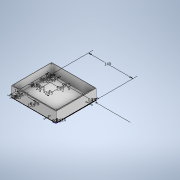
# Autodesk Inventor part: Couvercle inférieur
Saved by Autodesk Inventor 2020 (Build 240168000, 168)
## iProperties
Created: 2020-01-03
Part Number: Couvercle inférieur
Material: Générique
Document SubType Name: Modeling
Designer: Manuel Enzo
Density: 1 g/cm^3
Appearance: Par défaut
Author: Manuel Enzo
Autodesk Inventor part; units mm, degrees
ref_plane "YZ Plane" through (0, 0, 0) normal (1, 0, 0) x (0, 1, 0)
ref_plane "XZ Plane" through (0, 0, 0) normal (0, 1, 0) x (-1, 0, 0)
ref_plane "XY Plane" through (0, 0, 0) normal (0, 0, 1) x (1, 0, 0)
sketch "Esquisse1" plane through (0, 0, 0) normal (0, 1, 0) x (-1, 0, 0)
  line L0 (0, 0) -> (140, 0)
  line L1 (140, 0) -> (140, -126)
  line L2 (140, -126) -> (0, -126)
  line L3 (0, -126) -> (0, 0)
  line L4 (1, -1) -> (139, -1)
  line L5 (139, -1) -> (139, -125)
  line L6 (139, -125) -> (1, -125)
  line L7 (1, -125) -> (1, -1)
  line L8 (138, -2) -> (2, -2)
  line L9 (2, -2) -> (2, -124)
  line L10 (2, -124) -> (138, -124)
  line L11 (138, -124) -> (138, -2)
  circle A0 centre (135.5, -4.5) radius 2.5
  circle A1 centre (135.5, -4.5) radius 0.75
  circle A2 centre (135.5, -4.5) radius 1.5
  circle A3 centre (135.5, -121.5) radius 2.5
  circle A4 centre (135.5, -121.5) radius 1.5
  circle A5 centre (135.5, -121.5) radius 0.75
  circle A6 centre (4.5, -121.5) radius 2.5
  circle A7 centre (4.5, -121.5) radius 1.5
  circle A8 centre (4.5, -121.5) radius 0.75
  circle A9 centre (4.5, -4.5) radius 2.5
  circle A10 centre (4.5, -4.5) radius 1.5
  circle A11 centre (4.5, -4.5) radius 0.75
  circle A12 centre (135.25, -93.5) radius 2.5
  circle A13 centre (135.25, -93.5) radius 0.25
  circle A14 centre (87.25, -99.5) radius 2.5
  circle A15 centre (87.25, -99.5) radius 0.25
  circle A16 centre (135.25, -17.5) radius 2.5
  circle A17 centre (135.25, -17.5) radius 0.25
  circle A18 centre (87.25, -17.5) radius 2.5
  circle A19 centre (87.25, -17.5) radius 0.25
  circle A20 centre (119.75, -69) radius 2.5
  circle A21 centre (119.75, -69) radius 0.25
  circle A22 centre (91.75, -69) radius 2.5
  circle A23 centre (91.75, -69) radius 0.25
  point P0 (0, -11)
  point P1 (0, -19)
  point P2 (0, -26.5)
  point P3 (0, -34.5)
  point P4 (0, -40)
  point P5 (0, -49)
  point P6 (97.5, -53)
  point P7 (100, -50.5)
  point P8 (4.5, -2)
  point P9 (2, -4.5)
  point P10 (2, -121.5)
  point P11 (4.5, -124)
  point P12 (135.5, -124)
  point P13 (138, -121.5)
  point P14 (138, -4.5)
  point P15 (135.5, -2)
  dimension "d0" = 126
  dimension "d1" = 140
  dimension "d2" = 1
  dimension "d3" = 1
  dimension "d4" = 1
  dimension "d5" = 1
  dimension "d6" = 1
  dimension "d8" = 1
  dimension "d10" = 124
  dimension "d11" = 1
  dimension "d12" = 1
  dimension "d13" = 0.75
  dimension "d14" = 5
  dimension "d15" = 2.5
  dimension "d16" = 2.5
  dimension "d17" = 0.75
  dimension "d18" = 1
  dimension "d19" = 5
  dimension "d20" = 2.5
  dimension "d21" = 2.5
  dimension "d22" = 0.75
  dimension "d23" = 1
  dimension "d24" = 5
  dimension "d25" = 2.5
  dimension "d26" = 2.5
  dimension "d27" = 5
  dimension "d28" = 1
  dimension "d29" = 0.75
  dimension "d30" = 2.5
  dimension "d31" = 2.5
  dimension "d114" = 2.25
  dimension "d115" = 5
  dimension "d118" = 2.25
  dimension "d119" = 5
  dimension "d134" = 2.25
  dimension "d135" = 5
  dimension "d150" = 2.25
  dimension "d151" = 5
  dimension "d166" = 2.25
  dimension "d167" = 5
  dimension "d170" = 2.25
  dimension "d171" = 5
  dimension "d176" = 2.75
  dimension "d177" = 15.5
  dimension "d178" = 15.5
  dimension "d179" = 50.75
  dimension "d180" = 18.25
  dimension "d181" = 46.25
  dimension "d182" = 2.75
  dimension "d183" = 50.75
  dimension "d184" = 30.5
  dimension "d185" = 24.5
  dimension "d186" = 55
  dimension "d187" = 55
  constraints: 24 centre point, 24 end point, 14 coincident, 6 parallel, 3 horizontal, 3 perpendicular
  measures "d0" distance between parallel lines of L0 L2
  measures "d1" distance between parallel lines of L3 L1
  measures "d2" distance between parallel lines of L5 L11
  measures "d3" distance between parallel lines of L10 L6
  measures "d4" distance between parallel lines of L7 L9
  measures "d5" distance between parallel lines of L8 L4
  measures "d6" distance between parallel lines of L3 L7
  measures "d8" distance between parallel lines of L6 L2
  measures "d10" distance of L6.end L4.start
  measures "d11" distance between parallel lines of L1 L5
  measures "d12" radial gap between concentric circles of A0 A2
  measures "d13" radial gap between concentric circles of A2 A1
  measures "d14" diameter of A0
  measures "d15" distance from line of L11 A0.centre
  measures "d16" distance from line of L8 A0.centre
  measures "d17" radial gap between concentric circles of A4 A5
  measures "d18" radial gap between concentric circles of A4 A3
  measures "d19" diameter of A3
  measures "d20" distance from line of A3.centre L11
  measures "d21" distance from line of A3.centre L10
  measures "d22" radial gap between concentric circles of A7 A8
  measures "d23" radial gap between concentric circles of A6 A7
  measures "d24" diameter of A6
  measures "d25" distance from line of A6.centre L10
  measures "d26" distance from line of A8.centre L9
  measures "d27" diameter of A9
  measures "d28" radial gap between concentric circles of A9 A10
  measures "d29" radial gap between concentric circles of A11 A10
  measures "d30" distance from line of L9 A10.centre
  measures "d31" distance from line of L8 A9.centre
  measures "d114" radial gap between concentric circles of A12 A13
  measures "d115" diameter of A12
  measures "d118" radial gap between concentric circles of A14 A15
  measures "d119" diameter of A14
  measures "d134" radial gap between concentric circles of A16 A17
  measures "d135" diameter of A16
  measures "d150" radial gap between concentric circles of A18 A19
  measures "d151" diameter of A18
  measures "d166" radial gap between concentric circles of A20 A21
  measures "d167" diameter of A20
  measures "d170" radial gap between concentric circles of A22 A23
  measures "d171" diameter of A22
  measures "d176" distance from line of L11 A16.centre
  measures "d177" distance from line of L8 A17.centre
  measures "d178" distance from line of L8 A18.centre
  measures "d179" distance from line of L11 A18.centre
  measures "d180" distance from line of L11 A20.centre
  measures "d181" distance from line of L11 A23.centre
  measures "d182" distance from line of L11 A13.centre
  measures "d183" distance from line of L11 A15.centre
  measures "d184" distance from line of L10 A13.centre
  measures "d185" distance from line of L10 A14.centre
  measures "d186" distance from line of L10 A22.centre
  measures "d187" distance from line of L10 A20.centre
extrude "Extrusion1" add sketch "Esquisse1" along normal blind 2 contours L11 A0 L8 | A0 L11 A3 L10 A6 L9 A9 L8 | A9 L9 L8 | L11 L10 A3 | A6 L10 L9 | A13 | A15 | A17 | A19 | A21 | A23
extrude "Extrusion2" add sketch "Esquisse1" along normal blind 4 contours A12 | A14 | A16 | A18 | A20 | A22
extrude "Extrusion3" add sketch "Esquisse1" along normal blind 33.25 contours L4 L5 L6 L7 | A0 | A9 | A3 | A6 | A2 | A4 | A7 | A10
extrude "Extrusion4" cut sketch "Esquisse1" along normal blind 32.25 contours A2 | A4 | A7 | A10
extrude "Extrusion5" add sketch "Esquisse1" along normal blind 31.75 contours L0 L1 L2 L3
